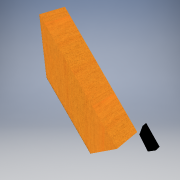
# Autodesk Inventor part: Angled Support Attachment
Saved by Autodesk Inventor 2016 (Build 200138000, 138)
## iProperties
Created: 2015-05-23
Part Number: Angled Support Attachment
Material: Generic
Document SubType Name: Modeling
Designer: Haden
Density: 1 g/cm^3
Appearance: Yellow Pine - Solid Stained Light Low Gloss
Author: Haden
Autodesk Inventor part; units mm, degrees
ref_plane "YZ Plane" through (0, 0, 0) normal (1, 0, 0) x (0, 1, 0)
ref_plane "XZ Plane" through (0, 0, 0) normal (0, 1, 0) x (-1, 0, 0)
ref_plane "XY Plane" through (0, 0, 0) normal (0, 0, 1) x (1, 0, 0)
sketch "Sketch1" plane through (0, 0, 0) normal (0, 0, 1) x (1, 0, 0)
  line L0 (0, 0) -> (0, 197.5656) construction
  line L1 (0, 197.5656) -> (716.8344, 914.4) construction
  line L2 (716.8344, 914.4) -> (914.4, 914.4) construction
  line L3 (914.4, 914.4) -> (0, 0) construction
  line L4 (481.8844, 679.45) -> (679.45, 679.45) construction
  line L5 (0, 742.3118) -> (0, 616.5882)
  line L6 (0, 616.5882) -> (209.5113, 407.0769)
  line L7 (209.5113, 407.0769) -> (272.3731, 469.9387)
  line L8 (272.3731, 469.9387) -> (0, 742.3118)
  point P0 (0, 679.45)
  dimension "d0" = 45
  dimension "d1" = 914.4
  dimension "d2" = 139.7
  dimension "d3" = 234.95
  dimension "d4" = 45
  dimension "d5" = 88.9
  constraints: 18 end point, 4 point on line, 3 perpendicular, 2 vertical, 1 collinear, 1 horizontal, 1 midpoint, 1 parallel
  measures "d0" angle of L0 L3
  measures "d1" distance from line of L2 L0.start
  measures "d2" distance between parallel lines of L3 L1
  measures "d3" distance between parallel lines of L2 L4
  measures "d4" angle of L8 L5
  measures "d5" distance between parallel lines of L8 L6
extrude "Extrusion1" add sketch "Sketch1" along normal blind 88.9
body "Solid1"
